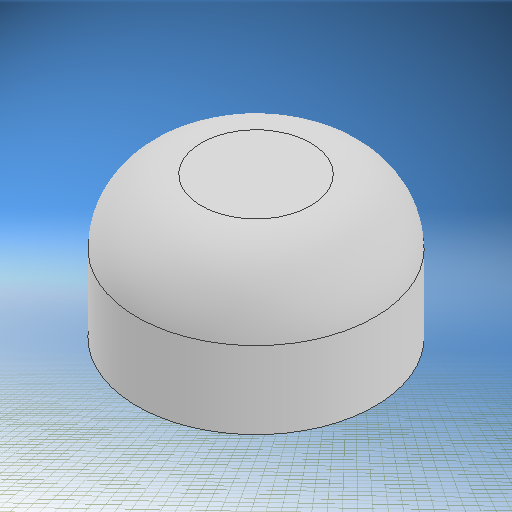
# Autodesk Inventor part: arm 2 cover_1
Saved by Autodesk Inventor 2025.1 (Build 291241000, 241)
## iProperties
Created: 2025-08-06
Part Number: arm 2 cover_1
Material: 일반
Document SubType Name: Modeling
Designer: joseph
Density: 1 g/cm^3
Appearance: 기본값
Author: joseph
Autodesk Inventor part; units mm, degrees
ref_plane "YZ Plane" through (0, 0, 0) normal (1, 0, 0) x (0, 1, 0)
ref_plane "XZ Plane" through (0, 0, 0) normal (0, 1, 0) x (-1, 0, 0)
ref_plane "XY Plane" through (0, 0, 0) normal (0, 0, 1) x (1, 0, 0)
sketch "스케치1" plane through (0, 0, 0) normal (0, 1, 0) x (-1, 0, 0)
  circle A0 centre (0, 0) radius 15.2
  circle A1 centre (0, 0) radius 18.5
  dimension "d0" = 30.4
  dimension "d1" = 37
  constraints: 2 centre point, 2 coincident
  measures "d0" diameter of A0
  measures "d1" diameter of A1
extrude "돌출1" add sketch "스케치1" along normal blind 20
sketch "스케치2" plane through (0, 20, 0) normal (0, 1, 0) x (1, 0, 0)
  circle A0 centre (0, 0) radius 18.5 projected
  circle A1 centre (0, 0) radius 15.2 projected
extrude "돌출2" add sketch "스케치2" along normal blind 2 contours A0 | A1
fillet "모깎기1" radius 10 2 edges at (15.2, 20, 0) (-18.5, 22, 0)
sketch "스케치3" plane through (0, 0, 0) normal (1, 0, 0) x (0, 1, 0)
  line L0 (0, -18.5) -> (0, 18.5) projected
  line L1 (4, 4) -> (0, 4)
  line L2 (0, 4) -> (0, -4)
  line L3 (0, -4) -> (4, -4)
  line L4 (4, -4) -> (4, 4)
  point P0 (0, 0)
  point P1 (0, 0)
  point P2 (0, 4)
  dimension "d7" = 4
  dimension "d8" = 8
  constraints: 8 end point, 2 midpoint, 2 parallel, 1 horizontal, 1 perpendicular
  measures "d7" distance of L3.end L2.end
  measures "d8" distance of L2.end L1.end
extrude "돌출3" cut sketch "스케치3" against normal through all
fillet "모깎기2" radius 2 4 edges at (-16.3633, 0, 4) (-16.3633, 4, -4) (-16.3633, 0, -4) (-16.3633, 4, 4)
